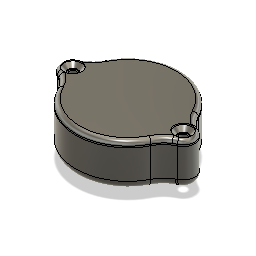
ultra7_airtag (Autodesk Fusion 360 design; units mm, degrees)
Autodesk Fusion 360 part; units mm, degrees
note: some values were not read from the file. Chosen so that the rebuilt part matches the saved one: which face or edge a step refers to. Set by a fixed rule: which sketch regions a step uses.
sketch "Base top" plane through (0, 0, 0) normal (0, 1, 0) x (1, 0, 0)
  circle A0 centre (0, 0) radius 3.4
  circle A1 centre (0, 0) radius 4.5
  line L0 (7, -9) -> (-7, -9)
  line L1 (-9, -7) -> (-9, 7)
  line L2 (-7, 9) -> (7, 9)
  line L3 (9, 7) -> (9, -7)
  line L4 (9, -9) -> (-9, 9) construction
  line L5 (-9, -9) -> (9, 9) construction
  arc A2 (-7, 9) -> (-9, 7) centre (-7, 7) ccw
  arc A3 (9, 7) -> (7, 9) centre (7, 7) ccw
  arc A4 (-9, -7) -> (-7, -9) centre (-7, -7) ccw
  arc A5 (7, -9) -> (9, -7) centre (7, -7) ccw
  line L6 (-45.2707, 0) -> (51.8354, 0) construction
  circle A6 centre (-5.842, 0) radius 1.8288
  line L7 (0, 0) -> (0, 17.1972) construction
  circle A7 centre (5.842, 0) radius 1.8288
  dimension "d1" = 6.8
  dimension "d2" = 9
  dimension "d3" = 18
  dimension "d4" = 18
  dimension "d5" = 2
  dimension "d6" = 2
  dimension "d7" = 2
  dimension "d8" = 2
  dimension "d9" = 3.6576
  dimension "d10" = 5.842
  constraint coincident A0.centre A1.centre
  constraint horizontal L0
  constraint perpendicular L0 L1
  constraint parallel L0 L2
  constraint parallel L1 L3
  constraint coincident L4 A0.centre
  constraint coincident L5 A0.centre
  constraint coincident L4.end L2
  constraint coincident L4.end L1
  constraint tangent L2 A2
  constraint tangent L1 A2
  constraint coincident L5.end L2
  constraint coincident L5.end L3
  constraint tangent L2 A3
  constraint tangent L3 A3
  constraint coincident L5.start L1
  constraint coincident L5.start L0
  constraint tangent L1 A4
  constraint tangent L0 A4
  constraint coincident L4.start L0
  constraint coincident L4.start L3
  constraint tangent L0 A5
  constraint tangent L3 A5
  constraint horizontal L6
  constraint coincident A0.centre L6
  constraint coincident L6 A6.centre
  constraint perpendicular L6 L7
  constraint symmetric A6 L7 A7
  measures "d1" diameter of A0
  measures "d2" diameter of A1
  measures "d3" distance of L4.end L5.end
  measures "d4" distance of L5.start L4.end
  measures "d5" radius of A2
  measures "d6" radius of A3
  measures "d7" radius of A4
  measures "d8" radius of A5
  measures "d9" diameter of A6
  measures "d10" distance of A0.centre A6.centre
extrude "Extrude1" add sketch "Base top" against normal blind 5 contours A1 A6 A7 | L0 L1 L2 L3 A2 A3 A4 A5 makes body 1
extrude "Extrude2" cut sketch "Base top" against normal blind 3 contours A1 A7 | A1 A6 A7 | A1 A6 picked at (5.2548, -0.6448) picked at (-4.3316, -0.2587) bodies 1
sketch "Tag top" plane through (0, 0, 0) normal (0, 1, 0) x (-1, 0, 0)
  arc A0 (9, 7) -> (7, 9) centre (7, 7) ccw
  line L0 (7, 9) -> (-7, 9)
  arc A1 (-7, 9) -> (-9, 7) centre (-7, 7) ccw
  line L1 (-9, 7) -> (-9, -7)
  arc A2 (-9, -7) -> (-7, -9) centre (-7, -7) ccw
  line L2 (-7, -9) -> (7, -9)
  arc A3 (7, -9) -> (9, -7) centre (7, -7) ccw
  line L3 (9, -7) -> (9, 7)
  circle A4 centre (0, 4) radius 13.25
  circle A5 centre (0, 4) radius 16
  circle A6 centre (0, 4) radius 18
  arc A7 (4.3679, 1.0824) -> (-4.3679, 1.0824) centre (0, 0) ccw
  arc A8 (4.3679, -1.0824) -> (4.3679, 1.0824) centre (5.842, 0) ccw
  arc A9 (-4.3679, -1.0824) -> (4.3679, -1.0824) centre (0, 0) ccw
  arc A10 (-4.3679, 1.0824) -> (-4.3679, -1.0824) centre (-5.842, 0) ccw
  line L4 (0, 4) -> (-38.6067, 4) construction
  line L5 (0, 0) -> (0, 25.9818) construction
  circle A11 centre (-19, 4) radius 1.25
  circle A12 centre (-19, 4) radius 2.85 construction
  circle A13 centre (-19, 4) radius 4
  circle A14 centre (19, 4) radius 4
  circle A15 centre (19, 4) radius 1.25
  dimension "d22" = 26.5
  dimension "d23" = 32
  dimension "d32" = 2.5
  dimension "d33" = 5.7
  dimension "d35" = 8
  dimension "d62" = 4
  dimension "d63" = 19
  constraint perpendicular L4 L5
  constraint coincident L4 A11.centre
  constraint concentric A11 A12
  constraint concentric A11 A13
  constraint symmetric L5 A11 A15
  constraint symmetric L5 A13 A14
  constraint concentric A5 A6
  constraint coincident A7.centre A9.centre
  constraint horizontal L4
  constraint coincident A4.centre L5
  constraint coincident A4.centre A5.centre
  measures "d22" diameter of A4
  measures "d23" diameter of A5
  measures "d32" diameter of A11
  measures "d33" diameter of A12
  measures "d35" diameter of A13
  measures "d62" distance of A4.centre A7.centre
  measures "d63" distance of A4.centre A11.centre
extrude "Extrude4" add sketch "Tag top" against normal up to surface (5 mm away) contours A0 L0 A1 L1 L2 L3 A4 | A0 L0 A1 L1 L3 A4 | L2 A3 L3 A4 | L2 A4 | L1 A2 L2 A4 | A5 A14 | A5 A6 A14 A15 | A5 A13 A14 | A5 A6 A13 A14 | A5 A6 A13 A14 | A5 A13 | A5 A6 A11 A13 | A6 A14 A15 | A6 A11 A13 bodies 1
extrude "Extrude5" add sketch "Tag top" along normal blind 1.8 contours L2 A3 L3 A4 | L1 A2 L2 A4 | A5 A14 | A5 A6 A14 A15 | A5 A13 A14 | A5 A6 A13 A14 | A5 A6 A13 A14 | A5 A13 | A5 A6 A11 A13 | A6 A14 A15 | A6 A11 A13 bodies 1
extrude "Extrude6" add sketch "Tag top" along normal blind 6.2 from surface at 1.8 contours A5 A6 A14 A15 | A5 A6 A13 A14 | A5 A6 A13 A14 | A5 A6 A11 A13 | A6 A14 A15 | A6 A11 A13 bodies 1
extrude "Extrude7" add sketch "Tag top" along normal blind 2 from surface at 8 separate body contours A0 L0 A1 L1 L2 L3 A4 | A0 L0 A1 L1 L3 A4 | L2 A3 L3 A4 | L2 A4 | L1 A2 L2 A4 | A5 A14 | A5 A6 A14 A15 | A5 A13 A14 | A5 A6 A13 A14 | A5 A6 A13 A14 | A5 A13 | A5 A6 A11 A13 | A6 A14 A15 | A6 A11 A13 | A6 A15 | A6 A15 | A6 A11 | A6 A11 | A7 A8 A9 A10 makes body 2
fillet "Fillet2" radius 10 8 edges at (17.6053, 1.5, 0.251) (17.6053, 1.5, 7.749) (-17.6053, 1.5, 0.251) (-17.6053, 1.5, 7.749) (17.6053, 9, 0.251) (17.6053, 9, 7.749) (-17.6053, 9, 0.251) (-17.6053, 9, 7.749) on bodies 1 2
sketch "Upper tag top" plane through (0, 10, 0) normal (0, 1, 0) x (-1, 0, 0)
  circle A0 centre (0, 4) radius 16
  circle A1 centre (19, 4) radius 1.25
  circle A2 centre (-19, 4) radius 1.25
  arc A3 (-16.0545, -4.1396) -> (16.0545, -4.1396) centre (0, 4) ccw
  arc A4 (20.7068, 0.3824) -> (16.0545, -4.1396) centre (24.9737, -8.6616) ccw
  arc A5 (20.7068, 0.3824) -> (20.7068, 7.6176) centre (19, 4) ccw
  arc A6 (16.0545, 12.1396) -> (20.7068, 7.6176) centre (24.9737, 16.6616) ccw
  arc A7 (16.0545, 12.1396) -> (-16.0545, 12.1396) centre (0, 4) ccw
  arc A8 (-20.7068, 7.6176) -> (-16.0545, 12.1396) centre (-24.9737, 16.6616) ccw
  arc A9 (-20.7068, 7.6176) -> (-20.7068, 0.3824) centre (-19, 4) ccw
  arc A10 (-16.0545, -4.1396) -> (-20.7068, 0.3824) centre (-24.9737, -8.6616) ccw
  circle A11 centre (0, 4) radius 16
  circle A12 centre (0, 4) radius 14.5
  circle A13 centre (-19, 4) radius 1.25
  circle A14 centre (19, 4) radius 1.25
  arc A15 (-16.0545, -4.1396) -> (16.0545, -4.1396) centre (0, 4) ccw
  arc A16 (20.7068, 0.3824) -> (16.0545, -4.1396) centre (24.9737, -8.6616) ccw
  arc A17 (20.7068, 0.3824) -> (20.7068, 7.6176) centre (19, 4) ccw
  arc A18 (16.0545, 12.1396) -> (20.7068, 7.6176) centre (24.9737, 16.6616) ccw
  arc A19 (16.0545, 12.1396) -> (-16.0545, 12.1396) centre (0, 4) ccw
  arc A20 (-20.7068, 7.6176) -> (-16.0545, 12.1396) centre (-24.9737, 16.6616) ccw
  arc A21 (-20.7068, 7.6176) -> (-20.7068, 0.3824) centre (-19, 4) ccw
  arc A22 (-16.0545, -4.1396) -> (-20.7068, 0.3824) centre (-24.9737, -8.6616) ccw
  circle A23 centre (19, 4) radius 3
  circle A24 centre (-19, 4) radius 3
  point P0 (19, 4)
  point P1 (-19, 4)
  dimension "d85" = 6
  dimension "d86" = 6
  constraint concentric A0 A12
  constraint concentric A14 A23
  constraint concentric A21 A24
  measures "d85" diameter of A23
  measures "d86" diameter of A24
extrude "Extrude8" add sketch "Upper tag top" against normal blind 1 from surface at -2 contours A0 A11 bodies 2
extrude "Extrude12" cut sketch "Upper tag top" against normal blind 0.4 contours A24 | A23 | A1 A14 | A2 A13 bodies 2
sketch "Upper tag holes" plane through (0, 9.6, 0) normal (0, 1, 0) x (-1, 0, 0)
  circle A0 centre (19, 4) radius 3
  point P0 (19, 4)
  point P1 (-19, 4)
hole "Hole4" at (-19, 9.6, 4) direction (0, -1, 0) diameter 3.4 end through all countersink diameter 6 countersink angle 90 bodies 2
hole "Hole5" at (19, 9.6, 4) direction (0, -1, 0) diameter 3.4 end through all countersink diameter 6 countersink angle 90 bodies 2
fillet "Fillet3" radius 0.5 2 edges at (14.9172, 7, 9.7858) (13.5187, 7, -1.2434) on bodies 2
fillet "Fillet4" radius 3 8 edges at (23, -5, 4) (18.0037, -5, -1.4908) (0, -5, -14) (-18.0037, -5, -1.4908) (-23, -5, 4) (-18.0037, -5, 9.4908) (0, -5, 22) (18.0037, -5, 9.4908) on bodies 1
fillet "Fillet5" radius 1.5 8 edges at (18.0037, 10, 9.4908) (23, 10, 4) (18.0037, 10, -1.4908) (0, 10, -14) (-18.0037, 10, -1.4908) (-23, 10, 4) (-18.0037, 10, 9.4908) (0, 10, 22) on bodies 2
fillet "Fillet6" radius 0.5 1 edges at (14.9172, 8, 9.7858) on bodies 1
fillet "Fillet7" radius 1 1 edges at (12.3533, 1.8, 8.7914) on bodies 1
fillet "Fillet8" radius 1 1 edges at (14.9172, 1.8, -1.7858) on bodies 1
fillet "Fillet9" radius 1 1 edges at (12.3533, 0, -0.7914) on bodies 1
extrude "Extrude10" add sketch "Base top" against normal up to surface (5 mm away) separate body contours A1 A7 picked at (5.2548, -0.6448) makes body 3
extrude "Extrude11" add sketch "Base top" against normal blind 3 from surface at -5 contours A1 A7 | A1 A7 bodies 3
scale "Scale1" factor 0.95 about (5.842, 0, 0) bodies 3
fillet "Fillet10" radius 0.5 1 edges at (4.1046, -7.6, 0) on bodies 3
fillet "Fillet11" radius 0.5 2 edges at (6.383, 0, -1.651) (6.383, 0, 1.651) on bodies 3
equation "LidThickness = 2 mm"
equation "d38 = LidThickness"
named bodies: "Tag mount base", "Tag mount lid", "Tag mount locator pin"
